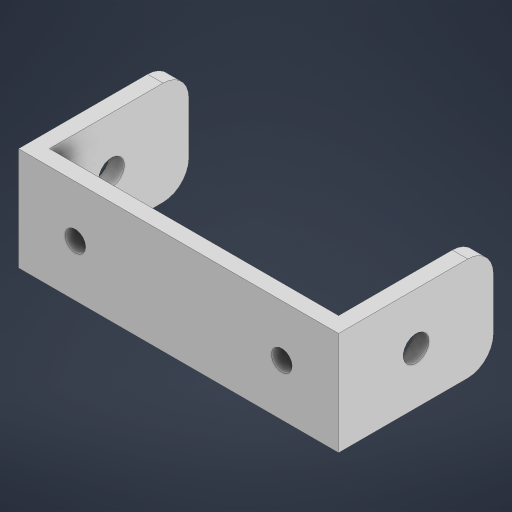
# Autodesk Inventor part: Aligner
Saved by Autodesk Inventor 2023 (Build 270158000, 158)
## iProperties
Created: 2023-11-08
Part Number: Aligner
Material: Generic
Document SubType Name: Modeling
Designer: Abhinav
Density: 1 g/cm^3
Appearance: Default
Author: Abhinav
Autodesk Inventor part; units mm, degrees
ref_plane "YZ Plane" through (0, 0, 0) normal (1, 0, 0) x (0, 1, 0)
ref_plane "XZ Plane" through (0, 0, 0) normal (0, 1, 0) x (-1, 0, 0)
ref_plane "XY Plane" through (0, 0, 0) normal (0, 0, 1) x (1, 0, 0)
sketch "Sketch1" plane through (0, 0, 0) normal (0, 1, 0) x (-1, 0, 0)
  line L0 (0, 0) -> (31, 0)
  line L1 (31, 0) -> (31, -30)
  line L2 (31, -30) -> (28, -30)
  line L3 (28, -30) -> (28, -3)
  line L4 (28, -3) -> (0, -3)
  line L5 (0, -3) -> (0, 0) construction
  line L6 (0, 0) -> (-31, 0)
  line L7 (-31, 0) -> (-31, -30)
  line L8 (-31, -30) -> (-28, -30)
  line L9 (-28, -30) -> (-28, -3)
  line L10 (-28, -3) -> (0, -3)
  dimension "d0" = 31
  dimension "d1" = 30
  dimension "d2" = 3
  dimension "d3" = 27
  constraints: 22 end point, 5 perpendicular, 4 symmetric about line, 1 horizontal
  measures "d0" distance of L0.start L0.end
  measures "d1" distance of L0.end L1.end
  measures "d2" distance of L1.end L2.end
  measures "d3" distance of L2.end L3.end
extrude "Extrusion1" add sketch "Sketch1" along normal blind 20
sketch "Sketch2" plane through (31, 0, 0) normal (1, 0, 0) x (0, 0, -1)
  line L0 (30, 0) -> (0, 0) construction
  line L1 (0, 0) -> (15, 0) construction
  line L2 (15, 0) -> (15, 10) construction
  circle A0 centre (15, 10) radius 2.5
  dimension "d6" = 15
  dimension "d7" = 10
  dimension "d8" = 5
  constraints: 4 end point, 1 centre point, 1 coincident, 1 midpoint, 1 vertical
  measures "d6" distance of L0.end L1.end
  measures "d7" distance of L1.end L2.end
  measures "d8" diameter of A0
extrude "Extrusion2" cut sketch "Sketch2" against normal blind 70
fillet "Fillet1" radius 5 4 edges at (29.5, 20, -30) (29.5, 0, -30) (-29.5, 0, -30) (-29.5, 20, -30)
sketch "Sketch3" plane through (28, 0, -3) normal (0, 0, -1) x (-1, 0, 0)
  line L0 (28, 0) -> (28, 10) construction
  line L1 (28, 10) -> (48, 10) construction
  circle A0 centre (48, 10) radius 2
  circle A1 centre (8, 10) radius 2
  dimension "d12" = 10
  dimension "d13" = 20
  dimension "d14" = 4
  constraints: 4 end point, 2 centre point, 1 coincident, 1 perpendicular, 1 symmetric about line, 1 vertical, 1 other
  measures "d12" distance of L0.start L0.end
  measures "d13" distance of L0.end L1.end
  measures "d14" diameter of A0
extrude "Extrusion3" cut sketch "Sketch3" against normal blind 10
body "Solid1"
